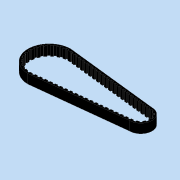
# Autodesk Inventor part: Pas zębaty 10 T5-315
Saved by Autodesk Inventor 2018 (Build 220112000, 112)
## iProperties
Created: 2019-01-25
Part Number: Pas zębaty 10 T5-315
Material: Ogólny
Document SubType Name: Modeling
Designer: Dawid
Density: 1 g/cm^3
Appearance: Anodowana - czarna
Author: Dawid
Autodesk Inventor part; units mm, degrees
ref_plane "YZ Plane" through (0, 0, 0) normal (1, 0, 0) x (0, 1, 0)
ref_plane "XZ Plane" through (0, 0, 0) normal (0, 1, 0) x (-1, 0, 0)
ref_plane "XY Plane" through (0, 0, 0) normal (0, 0, 1) x (1, 0, 0)
sketch "Szkic1" plane through (0, 0, 0) normal (0, 0, 1) x (1, 0, 0)
  circle A0 centre (0, 0) radius 9.525
  line L0 (0, 0) -> (-100, 0)
  circle A1 centre (-100, 0) radius 20.675
  line L1 (-100, 0) -> (-100, 20.675)
  line L2 (-100, 0) -> (-100, -20.675)
  line L3 (0, 0) -> (0, 9.525)
  line L4 (0, 0) -> (0, -9.525)
  line L5 (-100, 20.675) -> (0, 9.525)
  line L6 (-100, -20.675) -> (0, -9.525)
  line L7 (-100, 20.675) -> (-97.3, 20.675) construction
  line L8 (-100, -20.675) -> (-97.3, -20.675) construction
  line L9 (-100, 23.375) -> (0, 12.225)
  line L10 (-100, -23.375) -> (0, -12.225)
  arc A2 (-100, 23.375) -> (-100, -23.375) centre (-100, 0) ccw
  arc A3 (0, -12.225) -> (0, 12.225) centre (0, 0) ccw
  dimension "d1" = 100
  constraints: 22 end point, 8 point on circle, 4 centre point, 4 coincident, 3 horizontal, 1 parallel, 1 point on line, 1 vertical
  measures "d1" distance of L0.start L0.end
extrude "Wyciągnięcie proste1" add sketch "Szkic1" along normal blind 10
sketch "Szkic2" plane through (-95.4461, 20.1672, 0) normal (-0.1108, -0.9938, 0) x (0.9938, -0.1108, 0)
  line L0 (5, 0) -> (0, 0)
  line L1 (0, 10) -> (5, 10)
  line L2 (5, 0) -> (0, 0)
  line L3 (2.5, 0) -> (2.5, 10)
  line L4 (2.5, 0) -> (5, 0)
  line L5 (5, 0) -> (5, 10)
  line L6 (0, 10) -> (5, 10)
  line L7 (5, 10) -> (2.5, 10)
  line L8 (0, 0) -> (0, 10)
  point P0 (97.0931, 0)
  constraints: 18 end point, 1 midpoint
extrude "Wyciągnięcie proste2" cut sketch "Szkic2" against normal blind 1.2 contours L0 L3 L1 L5
pattern_linear "Szyk prostokątny1" count 19 spacing 5 along (0.9938, -0.1108, 0) of "Wyciągnięcie proste2"
sketch "Szkic3" plane through (-95.4461, -20.1672, 10) normal (-0.1108, 0.9938, 0) x (0.9938, 0.1108, 0)
  line L0 (5, 0) -> (0, 0)
  line L1 (2.5, 10) -> (5, 10)
  line L2 (0, 10) -> (2.5, 10)
  line L3 (2.5, 10) -> (5, 10)
  line L4 (5, 10) -> (5, 0)
  line L5 (5, 0) -> (0, 0)
  line L6 (2.5, 0) -> (2.5, 10)
  point P0 (97.0931, 10)
  dimension "d19" = 2.5
  constraints: 14 end point, 1 midpoint
  measures "d19" distance of L1.end L1.start
extrude "Wyciągnięcie proste3" cut sketch "Szkic3" against normal blind 1.2
pattern_linear "Szyk prostokątny2" count 19 spacing 5 along (0.9938, 0.1108, 0) of "Wyciągnięcie proste3"
sketch "Szkic4" plane through (0, 0, 0) normal (0, 0, -1) x (-1, 0, 0)
  arc A0 (0, 9.525) -> (0, -9.525) centre (0, 0) ccw projected
  line L0 (1.0312, -9.64) -> (0, -9.525) projected
  line L1 (0, 9.525) -> (1.0312, 9.64) projected
  line L2 (1.1834, -9.6225) -> (-1.3095, -9.4345)
  line L3 (-1.3095, -9.4345) -> (-3.7193, -8.7688)
  line L4 (-3.7193, -8.7688) -> (-5.8728, -7.4991)
  line L5 (-5.8728, -7.4991) -> (-7.6217, -5.7127)
  line L6 (-7.6217, -5.7127) -> (-8.8456, -3.5327)
  line L7 (-8.8456, -3.5327) -> (-9.4602, -1.1094)
  line L8 (-9.4602, -1.1094) -> (-9.423, 1.3903)
  line L9 (1.0312, 9.64) -> (-1.3594, 9.4275)
  line L10 (-1.3594, 9.4275) -> (1.0312, 9.64)
  line L11 (-1.3594, 9.4275) -> (-3.6728, 8.7884)
  line L12 (-3.6728, 8.7884) -> (-5.7529, 7.5914)
  line L13 (-5.7529, 7.5914) -> (-7.4679, 5.9124)
  line L14 (-7.4679, 5.9124) -> (-8.7087, 3.8581)
  line L15 (-8.7087, 3.8581) -> (-9.423, 1.3903)
  line L16 (-1.3095, -9.4345) -> (-3.7193, -8.7688)
  line L17 (-3.7193, -8.7688) -> (-4.0388, -9.9255)
  line L18 (-4.0388, -9.9255) -> (-1.6291, -10.5912)
  line L19 (-1.6291, -10.5912) -> (-1.3095, -9.4345)
  line L20 (-5.8728, -7.4991) -> (-7.6217, -5.7127)
  line L21 (-7.6217, -5.7127) -> (-8.4792, -6.5522)
  line L22 (-8.4792, -6.5522) -> (-6.7303, -8.3385)
  line L23 (-6.7303, -8.3385) -> (-5.8728, -7.4991)
  line L24 (-8.8456, -3.5327) -> (-9.4602, -1.1094)
  line L25 (-9.4602, -1.1094) -> (-10.6233, -1.4044)
  line L26 (-10.6233, -1.4044) -> (-10.0088, -3.8277)
  line L27 (-10.0088, -3.8277) -> (-8.8456, -3.5327)
  line L28 (-1.3594, 9.4275) -> (-3.6728, 8.7884)
  line L29 (-3.6728, 8.7884) -> (-3.9923, 9.9451)
  line L30 (-3.9923, 9.9451) -> (-1.6789, 10.5842)
  line L31 (-1.6789, 10.5842) -> (-1.3594, 9.4275)
  line L32 (-5.7529, 7.5914) -> (-7.4679, 5.9124)
  line L33 (-7.4679, 5.9124) -> (-8.3339, 6.797)
  line L34 (-8.3339, 6.797) -> (-6.619, 8.476)
  line L35 (-6.619, 8.476) -> (-5.7529, 7.5914)
  line L36 (-8.7087, 3.8581) -> (-9.423, 1.3903)
  line L37 (-9.423, 1.3903) -> (-10.5933, 1.729)
  line L38 (-10.5933, 1.729) -> (-9.879, 4.1968)
  line L39 (-9.879, 4.1968) -> (-8.7087, 3.8581)
  dimension "d25" = 2.5
  dimension "d26" = 2.5
  dimension "d27" = 2.5
  dimension "d28" = 2.5
  dimension "d29" = 2.5
  dimension "d30" = 2.5
  dimension "d31" = 2.5
  dimension "d32" = 2.4
  dimension "d33" = 2.4
  dimension "d34" = 2.4
  dimension "d35" = 2.4
  dimension "d36" = 2.4
  dimension "d37" = 2.4
  dimension "d38" = 1.2
  dimension "d39" = 1.2
  dimension "d40" = 1.2
  dimension "d41" = 1.2
  dimension "d42" = 1.2379
  dimension "d43" = 1.2184
  constraints: 76 end point, 13 parallel, 6 perpendicular, 2 collinear, 13 other
  measures "d25" distance of L2.start L2.end
  measures "d26" distance of L2.end L3.end
  measures "d27" distance of L3.end L4.end
  measures "d28" distance of L4.end L5.end
  measures "d29" distance of L5.end L6.end
  measures "d30" distance of L6.end L7.end
  measures "d31" distance of L7.end L8.end
  measures "d32" distance of L1.end L9.end
  measures "d33" distance of L9.end L1.end
  measures "d34" distance of L9.end L11.end
  measures "d35" distance of L11.end L12.end
  measures "d36" distance of L12.end L13.end
  measures "d37" distance of L13.end L14.end
  measures "d38" distance of L17.end L3.end
  measures "d39" distance of L21.end L5.end
  measures "d40" distance of L25.end L7.end
  measures "d41" distance of L11.end L29.end
  measures "d42" distance of L13.end L33.end
  measures "d43" distance of L8.end L37.end
extrude "Wyciągnięcie proste4" cut sketch "Szkic4" against normal up to next contours A0 L19 L18 L17 | L5 A0 | A0 L23 L22 L21 | A0 L27 L26 L25 | A0 L37 L38 L39 | A0 L33 L34 L35 | A0 L29 L30 L31
sketch "Szkic5" plane through (0, 0, 0) normal (0, 0, -1) x (-1, 0, 0)
  arc A0 (95.4461, -20.1672) -> (95.4461, 20.1672) centre (100, 0) ccw projected
  line L0 (92.9615, 19.8902) -> (95.4461, 20.1672) projected
  line L1 (95.4461, -20.1672) -> (92.9615, -19.8902) projected
  line L2 (92.9615, 19.8902) -> (95.4461, 20.1672)
  line L3 (95.4461, 20.1672) -> (97.9135, 20.5694)
  line L4 (97.9135, 20.5694) -> (100.4115, 20.6709)
  line L5 (100.4115, 20.6709) -> (102.8955, 20.4712)
  line L6 (102.8955, 20.4712) -> (105.3452, 19.9721)
  line L7 (105.3452, 19.9721) -> (107.7167, 19.1809)
  line L8 (107.7167, 19.1809) -> (109.9754, 18.1093)
  line L9 (109.9754, 18.1093) -> (112.0882, 16.7729)
  line L10 (112.0882, 16.7729) -> (114.0243, 15.1913)
  line L11 (114.0243, 15.1913) -> (115.82, 13.311)
  line L12 (115.82, 13.311) -> (117.3655, 11.2202)
  line L13 (117.3655, 11.2202) -> (118.6364, 8.952)
  line L14 (118.6364, 8.952) -> (119.6126, 6.5422)
  line L15 (119.6126, 6.5422) -> (120.2786, 4.029)
  line L16 (120.2786, 4.029) -> (120.6305, 1.3559)
  line L17 (92.9615, -19.8902) -> (95.4461, -20.1672)
  line L18 (95.4461, -20.1672) -> (97.9135, -20.5694)
  line L19 (97.9135, -20.5694) -> (100.4115, -20.6709)
  line L20 (100.4115, -20.6709) -> (102.9034, -20.4701)
  line L21 (102.9034, -20.4701) -> (105.3529, -19.97)
  line L22 (105.3529, -19.97) -> (107.7241, -19.178)
  line L23 (107.7241, -19.178) -> (109.9823, -18.1055)
  line L24 (109.9823, -18.1055) -> (112.1758, -16.7095)
  line L25 (112.1758, -16.7095) -> (114.1766, -15.0492)
  line L26 (114.1766, -15.0492) -> (115.9533, -13.1509)
  line L27 (115.9533, -13.1509) -> (117.4777, -11.0447)
  line L28 (117.4777, -11.0447) -> (118.7257, -8.7638)
  line L29 (118.7257, -8.7638) -> (119.6775, -6.3443)
  line L30 (119.6775, -6.3443) -> (120.3182, -3.8245)
  line L31 (120.3182, -3.8245) -> (120.6375, -1.2441)
  line L32 (120.6375, -1.2441) -> (120.6305, 1.3559)
  line L33 (120.2786, 4.029) -> (120.6305, 1.3559)
  line L34 (95.4461, 20.1672) -> (97.9135, 20.5694)
  line L35 (97.9135, 20.5694) -> (97.7407, 21.6298)
  line L36 (97.7407, 21.6298) -> (95.2733, 21.2276)
  line L37 (95.2733, 21.2276) -> (95.4461, 20.1672)
  line L38 (100.4115, 20.6709) -> (102.8955, 20.4712)
  line L39 (102.8955, 20.4712) -> (102.9917, 21.6674)
  line L40 (102.9917, 21.6674) -> (100.5076, 21.8671)
  line L41 (100.5076, 21.8671) -> (100.4115, 20.6709)
  line L42 (105.3452, 19.9721) -> (107.7167, 19.1809)
  line L43 (107.7167, 19.1809) -> (108.0964, 20.3193)
  line L44 (108.0964, 20.3193) -> (105.7249, 21.1104)
  line L45 (105.7249, 21.1104) -> (105.3452, 19.9721)
  line L46 (109.9754, 18.1093) -> (112.0882, 16.7729)
  line L47 (112.0882, 16.7729) -> (112.7297, 17.7871)
  line L48 (112.7297, 17.7871) -> (110.6169, 19.1235)
  line L49 (110.6169, 19.1235) -> (109.9754, 18.1093)
  line L50 (114.0243, 15.1913) -> (115.82, 13.311)
  line L51 (115.82, 13.311) -> (116.6878, 14.1398)
  line L52 (116.6878, 14.1398) -> (114.8921, 16.0201)
  line L53 (114.8921, 16.0201) -> (114.0243, 15.1913)
  line L54 (117.3655, 11.2202) -> (118.6364, 8.952)
  line L55 (118.6364, 8.952) -> (119.6833, 9.5386)
  line L56 (119.6833, 9.5386) -> (118.4124, 11.8068)
  line L57 (118.4124, 11.8068) -> (117.3655, 11.2202)
  line L58 (119.6126, 6.5422) -> (120.2786, 4.029)
  line L59 (120.2786, 4.029) -> (121.4386, 4.3364)
  line L60 (121.4386, 4.3364) -> (120.7726, 6.8496)
  line L61 (120.7726, 6.8496) -> (119.6126, 6.5422)
  line L62 (120.6305, 1.3559) -> (120.6375, -1.2441)
  line L63 (120.6375, -1.2441) -> (121.8375, -1.2409)
  line L64 (121.8375, -1.2409) -> (121.8305, 1.3591)
  line L65 (121.8305, 1.3591) -> (120.6305, 1.3559)
  line L66 (120.3182, -3.8245) -> (119.6775, -6.3443)
  line L67 (119.6775, -6.3443) -> (120.8405, -6.64)
  line L68 (120.8405, -6.64) -> (121.4812, -4.1201)
  line L69 (121.4812, -4.1201) -> (120.3182, -3.8245)
  line L70 (118.7257, -8.7638) -> (117.4777, -11.0447)
  line L71 (117.4777, -11.0447) -> (118.5304, -11.6207)
  line L72 (118.5304, -11.6207) -> (119.7784, -9.3398)
  line L73 (119.7784, -9.3398) -> (118.7257, -8.7638)
  line L74 (115.9533, -13.1509) -> (114.1766, -15.0492)
  line L75 (114.1766, -15.0492) -> (115.0528, -15.8692)
  line L76 (115.0528, -15.8692) -> (116.8294, -13.9709)
  line L77 (116.8294, -13.9709) -> (115.9533, -13.1509)
  line L78 (112.1758, -16.7095) -> (109.9823, -18.1055)
  line L79 (109.9823, -18.1055) -> (110.6267, -19.1178)
  line L80 (110.6267, -19.1178) -> (112.8201, -17.7218)
  line L81 (112.8201, -17.7218) -> (112.1758, -16.7095)
  line L82 (107.7241, -19.178) -> (105.3529, -19.97)
  line L83 (105.3529, -19.97) -> (105.7331, -21.1082)
  line L84 (105.7331, -21.1082) -> (108.1043, -20.3161)
  line L85 (108.1043, -20.3161) -> (107.7241, -19.178)
  line L86 (102.9034, -20.4701) -> (100.4115, -20.6709)
  line L87 (100.4115, -20.6709) -> (100.5078, -21.867)
  line L88 (100.5078, -21.867) -> (102.9998, -21.6662)
  line L89 (102.9998, -21.6662) -> (102.9034, -20.4701)
  line L90 (97.9135, -20.5694) -> (95.4461, -20.1672)
  line L91 (95.4461, -20.1672) -> (95.253, -21.3516)
  line L92 (95.253, -21.3516) -> (97.7205, -21.7538)
  line L93 (97.7205, -21.7538) -> (97.9135, -20.5694)
  point P0 (0, 0)
  dimension "d46" = 2.5
  dimension "d47" = 2.5
  dimension "d48" = 2.5
  dimension "d49" = 2.4921
  dimension "d50" = 2.5
  dimension "d51" = 2.5
  dimension "d52" = 2.5
  dimension "d53" = 2.5
  dimension "d54" = 2.5
  dimension "d55" = 2.6
  dimension "d56" = 2.6
  dimension "d57" = 2.6
  dimension "d58" = 2.6
  dimension "d59" = 2.6
  dimension "d61" = 2.5
  dimension "d62" = 2.5
  dimension "d63" = 2.5
  dimension "d64" = 2.5
  dimension "d65" = 2.5
  dimension "d66" = 2.5
  dimension "d67" = 2.5
  dimension "d68" = 2.6
  dimension "d69" = 2.6
  dimension "d70" = 2.6
  dimension "d71" = 2.6
  dimension "d72" = 2.6
  dimension "d73" = 2.6
  dimension "d74" = 2.6
  dimension "d75" = 2.6
  dimension "d76" = 2.6
  dimension "d77" = 1.0743
  dimension "d78" = 1.2
  dimension "d79" = 1.2
  dimension "d80" = 1.2
  dimension "d81" = 1.2
  dimension "d82" = 1.2
  dimension "d83" = 1.2
  dimension "d84" = 1.2
  dimension "d85" = 1.2
  dimension "d86" = 1.2
  dimension "d87" = 1.2
  dimension "d88" = 1.2
  dimension "d89" = 1.2
  dimension "d90" = 1.2
  dimension "d91" = 1.2
  constraints: 184 end point, 37 equal length, 15 perpendicular, 30 other
  measures "d46" distance of L0.start L0.end
  measures "d47" distance of L0.end L3.end
  measures "d48" distance of L3.end L4.end
  measures "d49" distance of L4.end L5.end
  measures "d50" distance of L5.end L6.end
  measures "d51" distance of L6.end L7.end
  measures "d52" distance of L7.end L8.end
  measures "d53" distance of L8.end L9.end
  measures "d54" distance of L9.end L10.end
  measures "d55" distance of L10.end L11.end
  measures "d56" distance of L11.end L12.end
  measures "d57" distance of L12.end L13.end
  measures "d58" distance of L13.end L14.end
  measures "d59" distance of L14.end L15.end
  measures "d61" distance of L1.end L1.start
  measures "d62" distance of L1.start L18.end
  measures "d63" distance of L18.end L19.end
  measures "d64" distance of L19.end L20.end
  measures "d65" distance of L20.end L21.end
  measures "d66" distance of L21.end L22.end
  measures "d67" distance of L22.end L23.end
  measures "d68" distance of L23.end L24.end
  measures "d69" distance of L24.end L25.end
  measures "d70" distance of L25.end L26.end
  measures "d71" distance of L26.end L27.end
  measures "d72" distance of L27.end L28.end
  measures "d73" distance of L28.end L29.end
  measures "d74" distance of L29.end L30.end
  measures "d75" distance of L30.end L31.end
  measures "d76" distance of L31.end L32.end
  measures "d77" distance of L35.end L3.end
  measures "d78" distance of L39.end L5.end
  measures "d79" distance of L43.end L7.end
  measures "d80" distance of L47.end L9.end
  measures "d81" distance of L51.end L11.end
  measures "d82" distance of L55.end L13.end
  measures "d83" distance of L59.end L15.end
  measures "d84" distance of L63.end L31.end
  measures "d85" distance of L67.end L29.end
  measures "d86" distance of L71.end L27.end
  measures "d87" distance of L75.end L25.end
  measures "d88" distance of L79.end L23.end
  measures "d89" distance of L83.end L21.end
  measures "d90" distance of L87.end L19.end
  measures "d91" distance of L91.end L1.start
extrude "Wyciągnięcie proste5" cut sketch "Szkic5" against normal up to next
